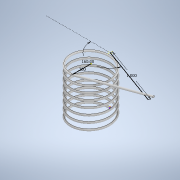
# Autodesk Inventor part: filiment
Saved by Autodesk Inventor 2020 (Build 240168000, 168)
## iProperties
Created: 2019-06-18
Part Number: filiment
Material: Generic
Document SubType Name: Modeling
Designer: ColinP
Density: 1 g/cm^3
Appearance: Default
Author: ColinP
Autodesk Inventor part; units mm, degrees
ref_plane "YZ Plane" through (0, 0, 0) normal (1, 0, 0) x (0, 1, 0)
ref_plane "XZ Plane" through (0, 0, 0) normal (0, 1, 0) x (-1, 0, 0)
ref_plane "XY Plane" through (0, 0, 0) normal (0, 0, 1) x (1, 0, 0)
sketch "Sketch1" plane through (0, 0, 0) normal (0, 1, 0) x (-1, 0, 0)
  line L0 (0, 0) -> (0, 7.62)
  dimension "d1" = 7.62
  constraints: 2 end point, 1 vertical
  measures "d1" distance of L0.start L0.end
sketch "Sketch3" plane through (0, 0, 0) normal (1, 0, 0) x (0, 1, 0)
  circle A0 centre (0, 7.6145) radius 0.381
  point P0 (0, 0)
  dimension "d3" = 0.762
  constraints: 1 centre point
  measures "d3" diameter of A0
sketch "Sketch2" plane through (0, 0, 0) normal (1, 0, 0) x (0, 1, 0)
  line L0 (0.8114, 0) -> (-0.5168, 0)
  point P0 (0, 0)
  constraints: 2 end point, 1 horizontal
coil "Coil1" sketch "Sketch3" operation add axis through (0, 0.8114, 0) along (0, -1, 0) pitch 2.54 turns 7.5 hand right
sketch "Sketch11" plane through (0, 0, 0) normal (0, 1, 0) x (-1, 0, 0)
  line L0 (0, 7.6145) -> (-23.8682, -1.0728)
  line L1 (0, 7.6145) -> (25.4, 7.6145) construction
  point P0 (0, 0)
  dimension "d21" = 25.4
  dimension "d22" = 160
  constraints: 4 end point, 1 equal length, 1 horizontal
  measures "d21" distance of L0.start L0.end
  measures "d22" angle of L0 L1
sketch "Sketch12" plane through (0, 0, 0) normal (0, 1, 0) x (-1, 0, 0)
  line L0 (0, -7.6145) -> (-23.8682, 1.0728)
  line L1 (0, -7.6145) -> (25.4, -7.6145) construction
  point P0 (0, 0)
  dimension "d23" = 25.4
  dimension "d24" = 160
  constraints: 4 end point, 1 equal length, 1 horizontal
  measures "d23" distance of L0.start L0.end
  measures "d24" angle of L1 L0
sketch "Sketch13" plane through (0, 0, 7.6145) normal (1, 0, 0) x (0, 0, -1)
  circle A0 centre (0, 0) radius 0.381 projected
  circle A1 centre (0, 0) radius 0.381
  point P0 (7.6145, 0)
  point P1 (0, 0.381)
  constraints: 1 centre point, 1 coincident, 1 vertical alignment
sketch "Sketch14" plane through (0, -19.05, -7.6145) normal (1, 0, 0) x (0, 0, -1)
  circle A0 centre (0, 0) radius 0.381 projected
  circle A1 centre (0, 0) radius 0.381
  point P0 (-7.6145, 19.05)
  point P1 (0, 0.381)
  constraints: 1 centre point, 1 coincident, 1 vertical alignment
sweep "Sweep5" add profiles "Sketch13" path "Sketch11"
body "Solid1"
